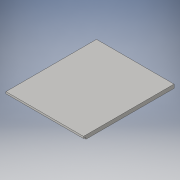
# Autodesk Inventor part: Horizontal Shelf with Lights Left
Saved by Autodesk Inventor 2016 (Build 200138000, 138)
## iProperties
Created: 2017-10-30
Part Number: Horizontal Shelf with Lights Left
Material: Generic
Document SubType Name: Modeling
Designer: mathaetaes
Density: 1 g/cm^3
Appearance: Default
Author: mathaetaes
Autodesk Inventor part; units mm, degrees
ref_plane "YZ Plane" through (0, 0, 0) normal (1, 0, 0) x (0, 1, 0)
ref_plane "XZ Plane" through (0, 0, 0) normal (0, 1, 0) x (-1, 0, 0)
ref_plane "XY Plane" through (0, 0, 0) normal (0, 0, 1) x (1, 0, 0)
sketch "Sketch1" plane through (0, 0, 0) normal (0, 1, 0) x (-1, 0, 0)
  line L0 (198.4375, -231.775) -> (-198.4375, -231.775)
  line L1 (-198.4375, -231.775) -> (-198.4375, 231.775)
  line L2 (-198.4375, 231.775) -> (198.4375, 231.775)
  line L3 (198.4375, 231.775) -> (198.4375, -231.775)
  line L4 (0, -324.485) -> (0, 324.485) projected
  line L5 (277.8125, 0) -> (-277.8125, 0) projected
  point P0 (0, 0)
  dimension "d0" = 396.875
  dimension "d1" = 463.55
  dimension "d4" = 198.4375
  dimension "d8" = 231.775
  constraints: 8 end point, 2 parallel, 1 horizontal, 1 perpendicular
  measures "d0" distance of L1.end L2.end
  measures "d1" distance of L0.end L1.end
  measures "d4" distance between parallel lines of L3 L4
  measures "d8" distance between parallel lines of L5 L0
extrude "Shelf Board" add sketch "Sketch1" along normal blind 19.05
sketch "Sketch3" plane through (0, 0, 0) normal (0, -1, 0) x (1, 0, 0)
  line L0 (-198.4375, 231.775) -> (198.4375, 231.775) projected
  line L1 (-128.5875, 231.775) -> (-90.4875, 231.775)
  line L2 (-90.4875, 231.775) -> (-90.4875, -180.975)
  line L3 (-90.4875, -180.975) -> (-128.5875, -180.975)
  line L4 (-128.5875, -180.975) -> (-128.5875, 231.775)
  line L5 (-198.4375, -231.775) -> (198.4375, -231.775) projected
  line L6 (-198.4375, 231.775) -> (-198.4375, -231.775) projected
  line L7 (-14.2875, 231.775) -> (23.8125, 231.775)
  line L8 (23.8125, 231.775) -> (23.8125, -180.975)
  line L9 (23.8125, -180.975) -> (-14.2875, -180.975)
  line L10 (-14.2875, -180.975) -> (-14.2875, 231.775)
  line L11 (198.4375, 231.775) -> (-198.4375, 231.775) projected
  line L12 (100.0125, 231.775) -> (138.1125, 231.775)
  line L13 (138.1125, 231.775) -> (138.1125, -180.975)
  line L14 (138.1125, -180.975) -> (100.0125, -180.975)
  line L15 (100.0125, -180.975) -> (100.0125, 231.775)
  line L16 (198.4375, 231.775) -> (198.4375, -231.775) projected
  line L17 (-198.4375, 231.775) -> (198.4375, 231.775)
  line L18 (198.4375, 231.775) -> (198.4375, 219.075)
  line L19 (198.4375, 219.075) -> (-198.4375, 219.075)
  line L20 (-198.4375, 219.075) -> (-198.4375, 231.775)
  point P0 (0, 0)
  dimension "d11" = 50.8
  dimension "d12" = 38.1
  dimension "d13" = 69.85
  dimension "d20" = 12.7
  dimension "d22" = 396.875
  dimension "d25" = 76.2
  dimension "d26" = 76.2
  dimension "d27" = 60.325
  constraints: 32 end point, 8 parallel, 6 collinear, 4 horizontal, 4 perpendicular, 2 point on line
  measures "d11" distance between parallel lines of L3 L5
  measures "d12" distance of L2.end L3.end
  measures "d13" distance between parallel lines of L4 L6
  measures "d20" distance of L17.end L18.end
  measures "d22" distance of L5.start L5.end
  measures "d25" distance between parallel lines of L2 L10
  measures "d26" distance between parallel lines of L8 L15
  measures "d27" distance between parallel lines of L13 L16
extrude "Light Stop Dados" cut sketch "Sketch3" against normal blind 9.525 contours L0 L4 L19 L6 | L0 L2 L19 L4 | L0 L10 L19 L2 | L19 L2 L3 L4 | L0 L8 L19 L10 | L0 L15 L19 L8 | L19 L8 L9 L10 | L19 L13 L0 L16 | L0 L13 L19 L15 | L13 L14 L15 L19
equation "\"d4\" = 0.5 * d0"
equation "\"d8\" = 0.5 * d1"
body "Solid1"
